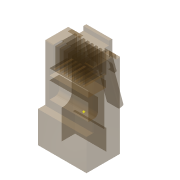
# Autodesk Inventor part: Part29
Saved by Autodesk Inventor 2022 (Build 260153000, 153)
## iProperties
Created: 2011-07-13
Part Number: Part29
Material: LCP Plastic
Document SubType Name: Modeling
Designer: manolis
Mass: 2.20824 g
Surface Area: 19.9866 cm^2
Volume: 1.35808 cm^3
Density: 1.626 g/cm^3
Appearance: Polycarbonate - Smoked
Author: manolis
Autodesk Inventor part; units mm, degrees
ref_plane "YZ Plane" through (0, 0, 0) normal (1, 0, 0) x (0, 1, 0)
ref_plane "XZ Plane" through (0, 0, 0) normal (0, 1, 0) x (-1, 0, 0)
sketch "Sketch1" plane through (0, 0, 0) normal (0, 0, 1) x (1, 0, 0)
  line L0 (-5.8, 3.25) -> (5.8, 3.25)
  line L1 (5.8, 3.25) -> (5.8, -3.25)
  line L2 (5.8, -3.25) -> (-5.8, -3.25)
  line L3 (-5.8, -3.25) -> (-5.8, 3.25)
  point P0 (0, 0)
  point P1 (0, 3.25)
  point P2 (-5.8, 0)
  dimension "d0" = 11.6
  dimension "d1" = 6.5
  constraints: 8 end point, 2 midpoint, 2 parallel, 1 horizontal, 1 horizontal alignment, 1 perpendicular, 1 vertical alignment
  measures "d0" distance of L1.end L2.end
  measures "d1" distance of L0.end L1.end
extrude "Extrusion1" add sketch "Sketch1" along normal blind 21
sketch "Sketch2" plane through (0, 0, 21) normal (0, 0, 1) x (1, 0, 0)
  line L0 (-5.8, 3.25) -> (5.8, 3.25) projected
  line L1 (-3.05, 3.25) -> (3.05, 3.25)
  line L2 (3.05, 3.25) -> (3.05, 4.0889)
  line L3 (3.05, 4.0889) -> (-3.05, 4.0889)
  line L4 (-3.05, 4.0889) -> (-3.05, 3.25)
  point P0 (0, 0)
  dimension "d4" = 6.1
  dimension "d5" = 11.6
  dimension "d6" = 2.75
  constraints: 8 end point, 2 parallel, 1 horizontal, 1 perpendicular, 1 point on line
  measures "d4" distance of L3.end L2.end
  measures "d5" distance of L0.start L0.end
  measures "d6" horizontal distance of L3.end L0.start
extrude "Extrusion2" add sketch "Sketch2" along normal blind 1 and the other way blind 2.4
ref_plane "Work Plane1" through (3.05, 4.0889, 18.6) normal (0, 0.258819, -0.9659258) x (-1, 0, 0)
sketch "Sketch3" plane through (3.05, 4.0889, 18.6) normal (0, 0.258819, -0.9659258) x (-1, 0, 0)
  line L0 (0, 0) -> (6.1, 0) projected
  line L1 (0, 0) -> (6.1, 0)
  line L2 (6.1, 0) -> (6.0967, -0.5)
  line L3 (6.0967, -0.5) -> (-0.0033, -0.5)
  line L4 (-0.0033, -0.5) -> (0, 0)
  point P0 (3.05, -8.7636)
  dimension "d14" = 6.1
  dimension "d17" = 0.5
  dimension "d22" = 6.1
  dimension "d28" = 0.5
  constraints: 8 end point, 1 horizontal
  measures "d14" distance of L0.start L0.end
  measures "d17" distance of L1.end L3.start
  measures "d22" distance of L3.start L3.end
  measures "d28" distance of L3.end L1.start
extrude "Extrusion3" add sketch "Sketch3" along normal blind 4 and the other way blind 0.75
sketch "Sketch4" plane through (3.05, 5.1241, 14.7363) normal (0, 0.258819, -0.9659258) x (-1, 0, 0)
  line L0 (6.1, 0) -> (6.0967, -0.5) projected
  line L1 (0, 0) -> (6.1, 0) projected
  line L2 (-0.0033, -0.5) -> (0, 0) projected
  line L3 (6.0967, -0.5) -> (-0.0033, -0.5) projected
  line L4 (1.4967, 0) -> (4.5967, 0)
  line L5 (4.5967, -0.5) -> (4.5967, 0.8)
  line L6 (4.5967, 0.8) -> (1.4967, 0.8)
  line L7 (1.4967, 0.8) -> (1.4967, -0.5)
  point P0 (3.05, -8.7636)
  dimension "d23" = 3.1
  dimension "d25" = 6.1
  dimension "d27" = 1.3
  constraints: 8 end point, 5 point on line, 2 parallel, 1 horizontal, 1 perpendicular
  measures "d23" distance of L6.end L5.end
  measures "d25" distance of L1.start L0.start
  measures "d27" distance of L5.start L5.end
extrude "Extrusion4" add sketch "Sketch4" along normal blind 10 and the other way blind 1 contours L5 L3 L7 L1 | L1 L7 L6 L5
fillet "Fillet1" radius 1 2 edges at (0.0033, 5.6381, 15.9093) (0.0033, 4.8653, 15.7022)
fillet "Fillet2" radius 0.2 8 edges at (0, 4.0889, 22) (5.8, 3.25, 10.5) (5.8, 0, 21) (-5.8, 3.25, 10.5) (-5.8, 0, 21) (0, -3.25, 21) (5.8, -3.25, 10.5) (-5.8, -3.25, 10.5)
sketch "Sketch5" plane through (-5.8, -3.05, 0) normal (-1, 0, 0) x (0, 0, 1)
  line L0 (21, 0) -> (21, 6.3) projected
  line L1 (21, 6.3) -> (20, 6.3)
  line L2 (20, 6.3) -> (20, 5.3)
  line L3 (20, 5.3) -> (21, 5.3)
  line L4 (21, 5.3) -> (21, 6.3)
  point P0 (0, 3.05)
  dimension "d35" = 1
  dimension "d36" = 1
  constraints: 8 end point, 2 parallel, 1 horizontal, 1 perpendicular
  measures "d35" distance of L3.end L2.end
  measures "d36" distance of L2.end L1.end
extrude "Extrusion5" cut sketch "Sketch5" against normal up to surface (2.75 mm away)
sketch "Sketch6" plane through (5.8, -3.05, 0) normal (1, 0, 0) x (0, 0, -1)
  line L0 (-20, 5.3) -> (-20, 6.1) projected
  line L1 (-20.8, 5.3) -> (-20, 5.3) projected
  line L2 (0, 6.3) -> (-21, 6.3) projected
  line L3 (-20, 5.3) -> (-21, 5.3)
  line L4 (-21, 5.3) -> (-21, 6.3)
  line L5 (-21, 6.3) -> (-20, 6.3)
  line L6 (-20, 6.3) -> (-20, 5.3)
  point P0 (0, 3.05)
  constraints: 8 end point, 2 parallel, 1 horizontal, 1 perpendicular
extrude "Extrusion6" cut sketch "Sketch6" against normal up to surface (2.75 mm away)
sketch "Sketch7" plane through (0, 0, 21) normal (0, 0, 1) x (1, 0, 0)
  line L0 (5.6, -3.05) -> (-5.6, -3.05) projected
  line L1 (-5.8, 2.25) -> (-5.8, -3.05) projected
  line L2 (-3.75, -3.25) -> (-3.75, -1.25)
  line L3 (-3.75, -1.25) -> (-3.25, -1.25)
  line L4 (-3.25, -1.25) -> (-3.25, -3.25)
  line L5 (-3.25, -3.25) -> (-3.25, -1.25)
  line L6 (-3.25, -1.25) -> (-3.75, -1.25)
  line L7 (-3.75, -1.25) -> (-3.75, -3.25)
  line L8 (-2.75, -3.25) -> (-2.75, -1.25)
  line L9 (-2.75, -1.25) -> (-2.25, -1.25)
  line L10 (-2.25, -1.25) -> (-2.25, -3.25)
  line L11 (-1.75, -3.25) -> (-1.75, -1.25)
  line L12 (-1.75, -1.25) -> (-1.25, -1.25)
  line L13 (-1.25, -1.25) -> (-1.25, -3.25)
  line L14 (-0.75, -3.25) -> (-0.75, -1.25)
  line L15 (-0.75, -1.25) -> (-0.25, -1.25)
  line L16 (-0.25, -1.25) -> (-0.25, -3.25)
  line L17 (0.25, -3.25) -> (0.25, -1.25)
  line L18 (0.25, -1.25) -> (0.75, -1.25)
  line L19 (0.75, -1.25) -> (0.75, -3.25)
  line L20 (1.25, -3.25) -> (1.25, -1.25)
  line L21 (1.25, -1.25) -> (1.75, -1.25)
  line L22 (1.75, -1.25) -> (1.75, -3.25)
  line L23 (2.25, -3.25) -> (2.25, -1.25)
  line L24 (2.25, -1.25) -> (2.75, -1.25)
  line L25 (2.75, -1.25) -> (2.75, -3.25)
  line L26 (3.25, -3.25) -> (3.25, -1.25)
  line L27 (3.25, -1.25) -> (3.75, -1.25)
  line L28 (3.75, -1.25) -> (3.75, -3.25)
  line L29 (5.8, -3.05) -> (5.8, 2.25) projected
  line L30 (-3.75, -1.25) -> (-3.25, -1.25)
  line L31 (-3.25, -1.25) -> (-3.25, -3.25)
  line L32 (-3.25, -3.25) -> (-3.75, -3.25)
  line L33 (-3.75, -3.25) -> (-3.75, -1.25)
  line L34 (-2.75, -1.25) -> (-2.25, -1.25)
  line L35 (-2.25, -1.25) -> (-2.25, -3.25)
  line L36 (-2.25, -3.25) -> (-2.75, -3.25)
  line L37 (-2.75, -3.25) -> (-2.75, -1.25)
  line L38 (-1.75, -1.25) -> (-1.25, -1.25)
  line L39 (-1.25, -1.25) -> (-1.25, -3.25)
  line L40 (-1.25, -3.25) -> (-1.75, -3.25)
  line L41 (-1.75, -3.25) -> (-1.75, -1.25)
  line L42 (-0.75, -1.25) -> (-0.25, -1.25)
  line L43 (-0.25, -1.25) -> (-0.25, -3.25)
  line L44 (-0.25, -3.25) -> (-0.75, -3.25)
  line L45 (-0.75, -3.25) -> (-0.75, -1.25)
  line L46 (0.25, -3.25) -> (0.75, -3.25)
  line L47 (0.75, -3.25) -> (0.75, -1.25)
  line L48 (0.75, -1.25) -> (0.25, -1.25)
  line L49 (0.25, -1.25) -> (0.25, -3.25)
  line L50 (1.25, -3.25) -> (1.75, -3.25)
  line L51 (1.75, -3.25) -> (1.75, -1.25)
  line L52 (1.75, -1.25) -> (1.25, -1.25)
  line L53 (1.25, -1.25) -> (1.25, -3.25)
  line L54 (2.25, -3.25) -> (2.75, -3.25)
  line L55 (2.75, -3.25) -> (2.75, -1.25)
  line L56 (2.75, -1.25) -> (2.25, -1.25)
  line L57 (2.25, -1.25) -> (2.25, -3.25)
  line L58 (3.25, -3.25) -> (3.75, -3.25)
  line L59 (3.75, -3.25) -> (3.75, -1.25)
  line L60 (3.75, -1.25) -> (3.25, -1.25)
  line L61 (3.25, -1.25) -> (3.25, -3.25)
  point P0 (0, 0)
  dimension "d43" = 0.5
  dimension "d44" = 0.5
  dimension "d45" = 0.5
  dimension "d46" = 0.5
  dimension "d47" = 2
  dimension "d48" = 0.5
  dimension "d49" = 0.5
  dimension "d50" = 2
  dimension "d51" = 0.5
  dimension "d52" = 0.5
  dimension "d53" = 2
  dimension "d54" = 0.5
  dimension "d55" = 0.5
  dimension "d56" = 2
  dimension "d57" = 0.5
  dimension "d58" = 0.5
  dimension "d59" = 2
  dimension "d60" = 0.5
  dimension "d61" = 0.5
  dimension "d62" = 2
  dimension "d63" = 0.5
  dimension "d65" = 2.05
  constraints: 118 end point, 17 parallel, 10 perpendicular, 8 horizontal
  measures "d43" distance of L2.end L3.end
  measures "d44" distance of L5.start L8.start
  measures "d45" distance of L8.end L9.end
  measures "d46" distance of L10.end L11.start
  measures "d47" distance of L11.start L11.end
  measures "d48" distance of L11.end L12.end
  measures "d49" distance of L13.end L14.start
  measures "d50" distance of L14.start L14.end
  measures "d51" distance of L14.end L15.end
  measures "d52" distance of L16.end L17.start
  measures "d53" distance of L17.start L17.end
  measures "d54" distance of L17.end L18.end
  measures "d55" distance of L19.end L20.start
  measures "d56" distance of L20.start L20.end
  measures "d57" distance of L20.end L21.end
  measures "d58" distance of L22.end L23.start
  measures "d59" distance of L23.start L23.end
  measures "d60" distance of L23.end L24.end
  measures "d61" distance of L25.end L26.start
  measures "d62" distance of L26.start L26.end
  measures "d63" distance of L26.end L27.end
  measures "d65" horizontal distance of L1.end L2.start
extrude "Extrusion7" cut sketch "Sketch7" against normal blind 5
sketch "Sketch8" plane through (-5.6, -3.25, 0) normal (0, -1, 0) x (1, 0, 0)
  line L0 (0, 0) -> (0, 20.8) projected
  line L1 (11.2, 20.8) -> (11.2, 0) projected
  line L2 (0.95, 15.7) -> (10.25, 15.7)
  line L3 (10.25, 15.7) -> (10.25, 14.2)
  line L4 (10.25, 14.2) -> (0.95, 14.2)
  line L5 (0.95, 14.2) -> (0.95, 15.7)
  point P0 (1.85, 16)
  point P1 (5.6, 0)
  dimension "d68" = 9.3
  dimension "d69" = 1.5
  dimension "d70" = 0.95
  dimension "d71" = 11.2
  dimension "d72" = 0.3
  constraints: 8 end point, 2 parallel, 1 horizontal, 1 perpendicular
  measures "d68" distance of L3.end L4.end
  measures "d69" distance of L2.end L3.end
  measures "d70" distance from line of L0 L2.start
  measures "d71" distance between parallel lines of L1 L0
  measures "d72" vertical distance of L2.start point (1.85, 16)
extrude "Extrusion8" cut sketch "Sketch8" against normal blind 4.2
sketch "Sketch9" plane through (-4.65, -3.25, 15.7) normal (1, 0, 0) x (0, 0, -1)
  line L0 (1.5, 0) -> (1.5, 4.2) projected
  line L1 (1.5, 0) -> (2.5, 0)
  line L2 (2.5, 0) -> (2.5, 2.3)
  line L3 (2.5, 0) -> (6.5, 0)
  line L4 (2.5, 2.3) -> (5.5, 2.3)
  line L5 (6.5, 1.3) -> (6.5, 0)
  line L6 (6.5, 0) -> (2.5, 0)
  line L7 (2.5, 0) -> (2.5, 2.3)
  arc A0 (6.5, 1.3) -> (5.5, 2.3) centre (5.5, 1.3) ccw
  point P0 (15.7, 3.25)
  dimension "d75" = 1
  dimension "d76" = 2.3
  dimension "d77" = 4
  dimension "d78" = 1
  constraints: 14 end point, 4 perpendicular, 2 parallel, 2 point on circle, 2 tangent, 1 centre point, 1 horizontal
  measures "d75" distance of L0.start L1.end
  measures "d76" distance of L1.end L2.end
  measures "d77" distance of L1.end L3.end
  measures "d78" radius of A0
extrude "Extrusion9" cut sketch "Sketch9" along normal up to surface (9.3 mm away)
sketch "Sketch10" plane through (-5.6, -3.25, 0) normal (0, -1, 0) x (1, 0, 0)
  line L0 (0, 0) -> (0, 20.8) projected
  line L1 (1.85, 21) -> (0, 21) projected
  line L2 (0, 21) -> (0, 7.5)
  line L3 (-0.2, 20.8) -> (-0.2, 0) projected
  line L4 (0, 7.5) -> (-0.2, 7.5)
  line L5 (11.4, 0) -> (11.4, 20.8) projected
  line L6 (-0.2, 7.5) -> (11.4, 7.5)
  line L7 (11.4, 7.5) -> (11.4, 0)
  line L8 (11.4, 0) -> (-0.2, 0)
  line L9 (-0.2, 0) -> (-0.2, 7.5)
  point P0 (5.6, 0)
  dimension "d81" = 13.5
  constraints: 12 end point, 2 parallel, 2 perpendicular, 2 point on line, 1 horizontal
  measures "d81" distance of L1.end L2.end
extrude "Extrusion10" add sketch "Sketch10" along normal blind 1.6 and the other way blind 2.1
sketch "Sketch11" plane through (-3.75, -3.05, 21) normal (1, 0, 0) x (0, 0, -1)
  line L0 (5.3, 4) -> (6.8, 4) projected
  line L1 (0.2, 4.2159) -> (12.0126, 4.2159)
  line L2 (16.0721, 4.5055) -> (0.2, 4.5055)
  line L3 (0.2, 4.5055) -> (0.2, 4.2159)
  line L4 (21, 4.5055) -> (21, 5.0204)
  line L5 (21, 5.0204) -> (16.0721, 5.0204)
  line L6 (16.0721, 5.0204) -> (16.0721, 4.5055)
  line L7 (14.0126, 1.8) -> (21, 1.8)
  line L8 (21, 1.8) -> (21, 4.5055)
  line L9 (16.0721, 4.5055) -> (14.0126, 4.5055)
  line L10 (14.0126, 2.2159) -> (14.0126, 1.8)
  arc A0 (14.0126, 2.2159) -> (12.0126, 4.2159) centre (12.0126, 2.2159) ccw
  point P0 (21, 3.05)
  dimension "d86" = 2
  constraints: 20 end point, 4 parallel, 2 horizontal, 2 point on circle, 2 tangent, 1 centre point, 1 perpendicular, 1 point on line
  measures "d86" radius of A0
extrude "Extrusion11" cut sketch "Sketch11" along normal up to surface (7.5 mm away)
fillet "Fillet3" radius 1.95 1 edges at (0, 4.0889, 18.6)
sketch "Sketch12" plane through (3.75, -3.25, 20.8) normal (0, -1, 0) x (1, 0, 0)
  line L0 (-7.5, 0.2) -> (-9.35, 0.2) projected
  line L1 (-6.5, 0.2) -> (-7, 0.2) projected
  line L2 (-5.5, 0.2) -> (-6, 0.2) projected
  line L3 (-4.5, 0.2) -> (-5, 0.2) projected
  line L4 (-3.5, 0.2) -> (-4, 0.2) projected
  line L5 (-2.5, 0.2) -> (-3, 0.2) projected
  line L6 (-1.5, 0.2) -> (-2, 0.2) projected
  line L7 (-0.5, 0.2) -> (-1, 0.2) projected
  line L8 (-7, 0.2) -> (-6.5, 0.2)
  line L9 (-6.5, 0.2) -> (-6.5, -4.8)
  line L10 (-6.5, -4.8) -> (-7, -4.8)
  line L11 (-7, -4.8) -> (-7, 0.2)
  line L12 (-6, 0.2) -> (-5.5, 0.2)
  line L13 (-5.5, 0.2) -> (-5.5, -4.8)
  line L14 (-5.5, -4.8) -> (-6, -4.8)
  line L15 (-6, -4.8) -> (-6, 0.2)
  line L16 (-5, -4.8) -> (-4.5, -4.8)
  line L17 (-4.5, -4.8) -> (-4.5, 0.2)
  line L18 (-4.5, 0.2) -> (-5, 0.2)
  line L19 (-5, 0.2) -> (-5, -4.8)
  line L20 (-4, -4.8) -> (-3.5, -4.8)
  line L21 (-3.5, -4.8) -> (-3.5, 0.2)
  line L22 (-3.5, 0.2) -> (-4, 0.2)
  line L23 (-4, 0.2) -> (-4, -4.8)
  line L24 (-3, -4.8) -> (-2.5, -4.8)
  line L25 (-2.5, -4.8) -> (-2.5, 0.2)
  line L26 (-2.5, 0.2) -> (-3, 0.2)
  line L27 (-3, 0.2) -> (-3, -4.8)
  line L28 (-2, -4.8) -> (-1.5, -4.8)
  line L29 (-1.5, -4.8) -> (-1.5, 0.2)
  line L30 (-1.5, 0.2) -> (-2, 0.2)
  line L31 (-2, 0.2) -> (-2, -4.8)
  line L32 (-1, -4.8) -> (-0.5, -4.8)
  line L33 (-0.5, -4.8) -> (-0.5, 0.2)
  line L34 (-0.5, 0.2) -> (-1, 0.2)
  line L35 (-1, 0.2) -> (-1, -4.8)
  point P0 (-3.75, -20.8)
  constraints: 56 end point, 14 parallel, 7 horizontal, 7 perpendicular
extrude "Extrusion12" add sketch "Sketch12" against normal up to surface (5.5 mm away)
sketch "Sketch13" plane through (3.25, -1.25, 21) normal (0, -1, 0) x (1, 0, 0)
  line L0 (0.5, -5) -> (0, -5)
  line L1 (0.5, 0) -> (0.5, -5)
  line L2 (-0.5, -5) -> (-1, -5)
  line L3 (-0.5, 0) -> (-0.5, -5)
  line L4 (-1, 0) -> (-0.5, 0)
  line L5 (-1, 0) -> (-1, -5)
  line L6 (-1.5, -5) -> (-2, -5)
  line L7 (-1.5, 0) -> (-1.5, -5)
  line L8 (-2, 0) -> (-1.5, 0)
  line L9 (-2, 0) -> (-2, -5)
  line L10 (-2.5, -5) -> (-3, -5)
  line L11 (-2.5, 0) -> (-2.5, -5)
  line L12 (-3, 0) -> (-2.5, 0)
  line L13 (-3, 0) -> (-3, -5)
  line L14 (-3.5, -5) -> (-4, -5)
  line L15 (-3.5, 0) -> (-3.5, -5)
  line L16 (-4, 0) -> (-3.5, 0)
  line L17 (-4, 0) -> (-4, -5)
  line L18 (-4.5, -5) -> (-5, -5)
  line L19 (-4.5, 0) -> (-4.5, -5)
  line L20 (-5, 0) -> (-4.5, 0)
  line L21 (-5, 0) -> (-5, -5)
  line L22 (-5.5, -5) -> (-6, -5)
  line L23 (-5.5, 0) -> (-5.5, -5)
  line L24 (-6, 0) -> (-5.5, 0)
  line L25 (-6, 0) -> (-6, -5)
  line L26 (-6.5, -5) -> (-7, -5)
  line L27 (-6.5, 0) -> (-6.5, -5)
  line L28 (-7, 0) -> (-6.5, 0)
  line L29 (-7, 0) -> (-7, -5)
  line L30 (0.5, 0) -> (0.5, -0.2)
  line L31 (0.5, -0.2) -> (0, -0.2)
  line L32 (0, -0.2) -> (0, -5)
  line L33 (0, -5) -> (0.5, -5)
  line L34 (0.5, -5) -> (0.5, -0.2)
  line L35 (-0.5, -0.2) -> (-1, -0.2)
  line L36 (-1, -0.2) -> (-1, -5)
  line L37 (-1, -5) -> (-0.5, -5)
  line L38 (-0.5, -5) -> (-0.5, -0.2)
  line L39 (-1.5, -0.2) -> (-2, -0.2)
  line L40 (-2, -0.2) -> (-2, -5)
  line L41 (-2, -5) -> (-1.5, -5)
  line L42 (-1.5, -5) -> (-1.5, -0.2)
  line L43 (-2.5, -0.2) -> (-3, -0.2)
  line L44 (-3, -0.2) -> (-3, -5)
  line L45 (-3, -5) -> (-2.5, -5)
  line L46 (-2.5, -5) -> (-2.5, -0.2)
  line L47 (-3.5, -0.2) -> (-4, -0.2)
  line L48 (-4, -0.2) -> (-4, -5)
  line L49 (-4, -5) -> (-3.5, -5)
  line L50 (-3.5, -5) -> (-3.5, -0.2)
  line L51 (-4.5, -0.2) -> (-5, -0.2)
  line L52 (-5, -0.2) -> (-5, -5)
  line L53 (-5, -5) -> (-4.5, -5)
  line L54 (-4.5, -5) -> (-4.5, -0.2)
  line L55 (-5.5, -0.2) -> (-6, -0.2)
  line L56 (-6, -0.2) -> (-6, -5)
  line L57 (-6, -5) -> (-5.5, -5)
  line L58 (-5.5, -5) -> (-5.5, -0.2)
  line L59 (-6.5, -0.2) -> (-7, -0.2)
  line L60 (-7, -0.2) -> (-7, -5)
  line L61 (-7, -5) -> (-6.5, -5)
  line L62 (-6.5, -5) -> (-6.5, -0.2)
  point P0 (-3.25, -21)
extrude "Extrusion13" cut sketch "Sketch13" against normal blind 3.2 contours L0 L32 L31 L1 | L2 L5 L35 L3 | L6 L9 L39 L7 | L10 L13 L43 L11 | L14 L17 L47 L15 | L18 L21 L51 L19 | L22 L25 L55 L23 | L26 L29 L59 L27
fillet "Fillet4" radius 0.3 4 edges at (0.0033, 8.4851, 5.2841) (1.5533, 7.8572, 5.1159) (-1.5467, 7.8572, 5.1159) (0.0033, 7.2294, 4.9476)
fillet "Fillet5" radius 0.3 12 edges at (-1.4589, 8.3775, 5.3462) (-1.5467, 5.6739, 15.3675) (-1.5467, 4.9225, 15.8966) (-1.5467, 7.1495, 10.2684) (-1.4589, 7.2915, 5.0552) (-1.5467, 5.8965, 9.9221) (1.4654, 8.3775, 5.3462) (1.5533, 5.6739, 15.3675) (1.5533, 4.9225, 15.8966) (1.5533, 7.1495, 10.2684) (1.4654, 7.2915, 5.0552) (1.5533, 5.8965, 9.9221)
equation "\"d6\" = -0.5 * d4 + 0.5 * d5"
equation "\"d44\" = d61"
equation "\"d46\" = d61"
equation "\"d49\" = d61"
equation "\"d52\" = d61"
equation "\"d55\" = d61"
equation "\"d58\" = d61"
equation "\"d70\" = -0.5 * d68 + 0.5 * d71"
body "Solid1"
